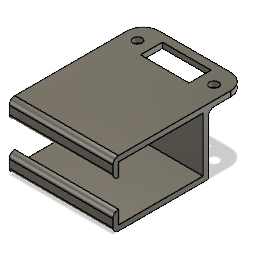
HDMI Port v2 (Autodesk Fusion 360 design; units mm, degrees)
Autodesk Fusion 360 part; units mm, degrees
sketch "Sketch1" plane through (0, 0, 0) normal (1, 0, 0) x (0, 0, -1)
  line L0 (0, 0) -> (-14, 0)
  line L1 (-14, 0) -> (-14, 2)
  line L2 (-14, 2) -> (0, 2)
  line L3 (0, 2) -> (0, 0)
  dimension "d1" = 14
  dimension "d2" = 2
  constraint horizontal L0
  constraint vertical L1
  constraint horizontal L2
  constraint vertical L3
  constraint coincident L0.start L3.end
  measures "d1" distance of L0.start L0.end
  measures "d2" distance of L0.start L2.end
extrude "Extrude1" add sketch "Sketch1" along normal blind 38
fillet "Fillet1" radius 5.9 4 edges at (0, 1, 14) (38, 1, 14) (38, 1, 0) (0, 1, 0)
sketch "Sketch2" plane through (0, 2, 0) normal (0, 1, 0) x (-1, 0, 0)
  arc A0 (-5.9, 0) -> (0, 5.9) centre (-5.9, 5.9) ccw
  line L0 (0, 5.9) -> (0, 8.1)
  arc A1 (0, 8.1) -> (-5.9, 14) centre (-5.9, 8.1) ccw
  line L1 (-5.9, 14) -> (-32.1, 14)
  arc A2 (-32.1, 14) -> (-38, 8.1) centre (-32.1, 8.1) ccw
  line L2 (-38, 8.1) -> (-38, 5.9)
  arc A3 (-38, 5.9) -> (-32.1, 0) centre (-32.1, 5.9) ccw
  line L3 (-32.1, 0) -> (-5.9, 0)
  line L4 (-19, 0) -> (-19, 14)
  line L5 (-19, 7) -> (-27.875, 7)
  line L6 (-27.875, 7) -> (-27.875, 3)
  line L7 (-27.875, 3) -> (-19, 3)
  line L8 (-19, 3) -> (-19, 7)
  line L9 (-27.875, 3) -> (-10.125, 3)
  line L10 (-10.125, 3) -> (-10.125, 11)
  line L11 (-10.125, 11) -> (-27.875, 11)
  line L12 (-27.875, 11) -> (-27.875, 3)
  line L13 (-10.125, 7) -> (-6.625, 7)
  circle A4 centre (-5, 7) radius 1.625
  line L14 (-27.875, 7) -> (-31.375, 7)
  circle A5 centre (-33, 7) radius 1.625
  dimension "d7" = 8.875
  dimension "d8" = 4
  dimension "d9" = 17.75
  dimension "d10" = 8
  dimension "d11" = 3.5
  dimension "d12" = 3.25
  dimension "d13" = 3.5
  dimension "d14" = 3.25
  constraint midpoint L3 L4.start
  constraint midpoint L1 L4.end
  constraint horizontal L5
  constraint vertical L6
  constraint horizontal L7
  constraint vertical L8
  constraint midpoint L4 L5.start
  constraint horizontal L9
  constraint vertical L10
  constraint horizontal L11
  constraint vertical L12
  constraint midpoint L10 L13.start
  constraint perpendicular L10 L13
  constraint coincident L13.end A4
  constraint perpendicular L6 L14
  constraint coincident L14.end A5
  measures "d7" distance of L5.start L5.end
  measures "d8" distance of L5.start L7.end
  measures "d9" distance of L6.end L9.end
  measures "d10" distance of L6.end L11.end
  measures "d11" distance of L13.start L13.end
  measures "d12" diameter of A4
  measures "d13" distance of L5.end L14.end
  measures "d14" diameter of A5
extrude "Extrude2" cut sketch "Sketch2" against normal blind 2 contours L4 L5 L6 L7 L8 L9 L12 | L4 L8 L9 L10 L11 | L4 L5 L11 L12 | A4 | A5
sketch "Sketch3" plane through (0, 2, 0) normal (0, 1, 0) x (-1, 0, 0)
  circle A0 centre (-33, 7) radius 1.625
  circle A1 centre (-5, 7) radius 1.625
  line L0 (-10.125, 3) -> (-27.875, 3)
  line L1 (-27.875, 3) -> (-27.875, 11)
  line L2 (-27.875, 11) -> (-10.125, 11)
  line L3 (-10.125, 11) -> (-10.125, 3)
  arc A2 (-5.9, 0) -> (0, 5.9) centre (-5.9, 5.9) ccw
  line L4 (0, 5.9) -> (0, 8.1)
  arc A3 (0, 8.1) -> (-5.9, 14) centre (-5.9, 8.1) ccw
  line L5 (-5.9, 14) -> (-32.1, 14)
  arc A4 (-32.1, 14) -> (-38, 8.1) centre (-32.1, 8.1) ccw
  line L6 (-38, 8.1) -> (-38, 5.9)
  arc A5 (-38, 5.9) -> (-32.1, 0) centre (-32.1, 5.9) ccw
  line L7 (-32.1, 0) -> (-5.9, 0)
  line L8 (-32.1, 14) -> (-32.1, 45)
  line L9 (-32.1, 45) -> (-38, 45)
  line L10 (-38, 45) -> (-38, 8.1)
  line L11 (-38, 8.1) -> (-32.1, 8.1)
  line L12 (-32.1, 8.1) -> (-32.1, 45)
  line L13 (-38, 45) -> (0, 45)
  line L14 (0, 45) -> (0, 8.1)
  line L15 (0, 8.1) -> (-38, 8.1)
  line L16 (-38, 8.1) -> (-38, 45)
  dimension "d17" = 31
  constraint coincident L5.end A4.start
  constraint perpendicular L5 L8
  constraint horizontal L9
  constraint vertical L10
  constraint horizontal L11
  constraint vertical L12
  constraint coincident A4.end L6.start
  constraint horizontal L13
  constraint vertical L14
  constraint horizontal L15
  constraint vertical L16
  constraint coincident L4.end A3.start
  measures "d17" distance of L5.end L8.end
extrude "Extrude3" add sketch "Sketch3" against normal blind 2 contours A4 L8 L9 L10 L12 L13 L16 | A3 L5 L8 L12 L13 L14
sketch "Sketch4" plane through (38, 0, 0) normal (1, 0, 0) x (0, 0, -1)
  line L0 (-5.9, 0) -> (-5.9, 2)
  line L1 (-5.9, 2) -> (-45, 2)
  line L2 (-45, 2) -> (-45, 0)
  line L3 (-45, 0) -> (-5.9, 0)
  line L4 (-45, 0) -> (-45, -5)
  line L5 (-45, -5) -> (-47, -5)
  line L6 (-47, -5) -> (-45, -5)
  line L7 (-45, -5) -> (-45, 2)
  line L8 (-45, 2) -> (-47, 2)
  line L9 (-47, 2) -> (-47, -5)
  line L10 (-45, 0) -> (-14, 0)
  line L11 (-14, 0) -> (-14, -20)
  line L12 (-14, -20) -> (-45, -20)
  line L13 (-45, -20) -> (-45, -15)
  line L14 (-45, -15) -> (-47, -15)
  line L15 (-47, -15) -> (-47, -22)
  line L16 (-47, -22) -> (-14, -22)
  line L17 (-14, -22) -> (-12, -22)
  line L18 (-12, -22) -> (-12, 0)
  line L19 (-12, 0) -> (-14, 0)
  line L20 (-14, 0) -> (-14, -22)
  dimension "d20" = 5
  dimension "d21" = 2
  dimension "d22" = 31
  dimension "d23" = 20
  dimension "d24" = 31
  dimension "d25" = 5
  dimension "d26" = 2
  dimension "d27" = 7
  dimension "d28" = 33
  dimension "d29" = 2
  dimension "d30" = 22
  constraint coincident L2.end L3.start
  constraint perpendicular L3 L4
  constraint perpendicular L4 L5
  constraint horizontal L6
  constraint vertical L7
  constraint horizontal L8
  constraint vertical L9
  constraint coincident L1.end L2.start
  constraint perpendicular L2 L10
  constraint perpendicular L10 L11
  constraint perpendicular L11 L12
  constraint perpendicular L12 L13
  constraint perpendicular L13 L14
  constraint perpendicular L14 L15
  constraint perpendicular L15 L16
  constraint horizontal L17
  constraint vertical L18
  constraint horizontal L19
  constraint vertical L20
  measures "d20" distance of L2.end L4.end
  measures "d21" distance of L4.end L5.end
  measures "d22" distance of L2.end L10.end
  measures "d23" distance of L10.end L11.end
  measures "d24" distance of L11.end L12.end
  measures "d25" distance of L12.end L13.end
  measures "d26" distance of L13.end L14.end
  measures "d27" distance of L14.end L15.end
  measures "d28" distance of L15.end L16.end
  measures "d29" distance of L16.end L17.end
  measures "d30" distance of L16.end L10.end
extrude "Extrude4" add sketch "Sketch4" against normal blind 38 contours L3 L11 L17 L18 L19 L20 | L2 L4 L5 L6 L7 L8 L9 | L12 L13 L14 L15 L16 L20
move_face "MoveFace1" by (0, 0, 2) 6 faces at (25.3333, -14.6667, 12) (25.3333, -6.6667, 14) (25.3333, -17.3333, 47) (25.3333, -18.3333, 45) (25.3333, -1.6667, 45) (25.3333, -0.3333, 47)
fillet "Fillet2" radius 2 1 edges at (19, 0, 14)
fillet "Fillet3" radius 2 1 edges at (19, 2, 49)
fillet "Fillet4" radius 2 1 edges at (19, -22, 49)
fillet "Fillet5" radius 2 2 edges at (19, -5, 49) (19, -15, 49)
equation "d7 = ( 17.75 / 2 ) * 1 mm"
equation "d9 = 8.875 mm * 2"
equation "d10 = 4.000 mm * 2"
